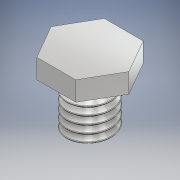
# Autodesk Inventor part: tornillo
Saved by Autodesk Inventor 2018 (Build 220112000, 112)
## iProperties
Created: 2019-11-12
Part Number: tornillo
Material: Generic
Document SubType Name: Modeling
Designer: Marie
Density: 1 g/cm^3
Appearance: Default
Author: Marie
Autodesk Inventor part; units mm, degrees
ref_plane "YZ Plane" through (0, 0, 0) normal (1, 0, 0) x (0, 1, 0)
ref_plane "XZ Plane" through (0, 0, 0) normal (0, 1, 0) x (-1, 0, 0)
sketch "Sketch1" plane through (0, 0, 0) normal (0, 0, 1) x (1, 0, 0)
  circle A0 centre (0, 0) radius 2.3
  dimension "d0" = 4.6
  constraints: 1 centre point, 1 coincident
  measures "d0" diameter of A0
extrude "Extrusion1" add sketch "Sketch1" along normal blind 5
ref_plane "Work Plane1" through (0, 0, 5) normal (0, 0, 1) x (1, 0, 0)
sketch "Sketch2" plane through (0, 0, 5) normal (0, 0, 1) x (1, 0, 0)
  line L0 (3.9923, 0) -> (1.9962, -3.4575)
  line L1 (1.9962, -3.4575) -> (-1.9962, -3.4575)
  line L2 (-1.9962, -3.4575) -> (-3.9923, 0)
  line L3 (-3.9923, 0) -> (-1.9962, 3.4575)
  line L4 (-1.9962, 3.4575) -> (1.9962, 3.4575)
  line L5 (1.9962, 3.4575) -> (3.9923, 0)
  point P0 (0, 0)
  point P1 (0, 0)
  constraints: 12 end point, 1 coincident, 13 other
extrude "Extrusion2" add sketch "Sketch2" along normal blind 2
thread "Thread1" size "M5x0.8" class "6g" standard "ANSI Metric M Profile" full length
sketch "Sketch4" plane through (0, 0, 5) normal (-1, 0, 0) x (0, 1, 0)
  line L0 (2.3, 0) -> (2.3, 5)
  line L1 (2.3, 5) -> (1.7068, 5)
  line L2 (1.7068, 5) -> (1.7068, 0)
  line L3 (1.7068, 0) -> (2.3, 0)
  line L4 (0, -3.4) -> (0, 6.4) projected
  constraints: 8 end point
revolve "Revolution1" cut sketch "Sketch4" angle 360 about axis through (0, 0, 5) along (0, 0, -1)
sketch "Sketch5" plane through (0, 0, 5) normal (-1, 0, 0) x (0, 1, 0)
  line L0 (2.3, 0) -> (2.3, 5)
  line L1 (2.3, 5) -> (1.7068, 5)
  line L2 (1.7068, 5) -> (1.7068, 0)
  line L3 (1.7068, 0) -> (2.3, 0)
  line L4 (0, -3.4) -> (0, 6.4) projected
  constraints: 8 end point
revolve "Revolution2" add sketch "Sketch5" angle 360 about axis through (0, 0, 5) along (0, 0, -1) separate body
sketch "Sketch3" plane through (0, 0, 5) normal (1, 0, 0) x (0, 0, -1)
  line L0 (-0.4668, -1.7475) -> (-0.4001, -1.7475) construction
  line L1 (0.0666, -2.2597) -> (-0.0001, -2.3878) construction
  line L2 (-0.8001, -2.3878) -> (-0.8668, -2.2597) construction
  line L3 (-0.3334, -1.7475) -> (-0.4001, -1.6194) construction
  line L4 (-0.4001, -1.6194) -> (-0.4668, -1.7475) construction
  line L5 (-0.8001, -2.3878) -> (-0.7334, -2.2597) construction
  line L6 (-0.3334, -1.7475) -> (-0.0668, -2.2597)
  line L7 (-0.8668, -2.2597) -> (-0.7334, -2.2597) construction
  arc A0 (-0.8668, -2.2597) -> (-0.8001, -2.3002) centre (-0.8001, -2.225) ccw construction
  line L8 (0.0666, -2.2597) -> (-0.0668, -2.2597) construction
  line L9 (-0.8001, -2.3878) -> (-0.8001, -2.2597) construction
  line L10 (-0.0001, -2.3878) -> (-0.0001, -2.2597) construction
  line L11 (-0.4001, -1.6194) -> (-0.4001, -1.707) construction
  line L12 (-0.8001, -2.3002) -> (-0.0001, -2.3002)
  arc A1 (-0.8001, -2.3002) -> (-0.7334, -2.2597) centre (-0.8001, -2.225) ccw
  line L13 (-0.0668, -2.2597) -> (-0.0001, -2.3878) construction
  line L14 (-0.7334, -2.2597) -> (-0.4668, -1.7475)
  line L15 (-0.0001, -0.0002) -> (-0.0001, 0.0177)
  line L16 (-0.0001, 0.0177) -> (-0.0001, -0.0002)
  line L17 (-0.0001, -0.0002) -> (0.0334, -0.0002)
  arc A2 (-0.0668, -2.2597) -> (-0.0001, -2.3002) centre (-0.0001, -2.225) ccw
  arc A3 (-0.0001, -2.3002) -> (0.0666, -2.2597) centre (-0.0001, -2.225) ccw construction
  arc A4 (-0.4001, -1.707) -> (-0.4668, -1.7475) centre (-0.4001, -1.7822) ccw
  arc A5 (-0.3334, -1.7475) -> (-0.4001, -1.707) centre (-0.4001, -1.7822) ccw
  line L18 (-0.4001, -1.707) -> (-0.4001, -1.7475) construction
  line L19 (-0.4001, -1.7475) -> (-0.3334, -1.7475) construction
  dimension "d8" = 55
  dimension "d9" = 0.1281
  dimension "d10" = 0.1281
  dimension "Sketch3_ThreadOffset" = 0
  dimension "Sketch3_MajorRadius" = 2.3
  dimension "d13" = 0.8
  dimension "Sketch3_MinorRadius" = 1.7068
  constraints: 40 end point, 12 point on circle, 10 parallel, 8 tangent, 6 centre point, 6 collinear, 2 midpoint, 2 point on line, 1 horizontal, 1 perpendicular, 3 other
  measures "d8" angle of L6 L14
  measures "d9" distance of L3.end L0.end
  measures "d10" distance of L1.end L10.end
  measures "Sketch3_ThreadOffset" distance between parallel lines of L15 L10
  measures "Sketch3_MajorRadius" distance from line of L12 L15.start
  measures "d13" distance from line of L1.end L9
  measures "Sketch3_MinorRadius" distance edge to line of A5 L17
coil "Coil1" sketch "Sketch3" operation cut axis through (0, 0, 5) along (0, 0, -1) pitch 0.8008 turns 8.241758 hand right bodies 2
equation "\"d8\" = d15"
equation "\"d9\" = 0.160083 * Sketch3_Pitch"
equation "\"d10\" = 0.160083 * Sketch3_Pitch"
equation "\"d13\" = Sketch3_Pitch"
equation "\"d15\" = 55deg"
equation "\"Sketch3_Pitch\" = 0.8"
body "Solid1"
body "Solid2"
